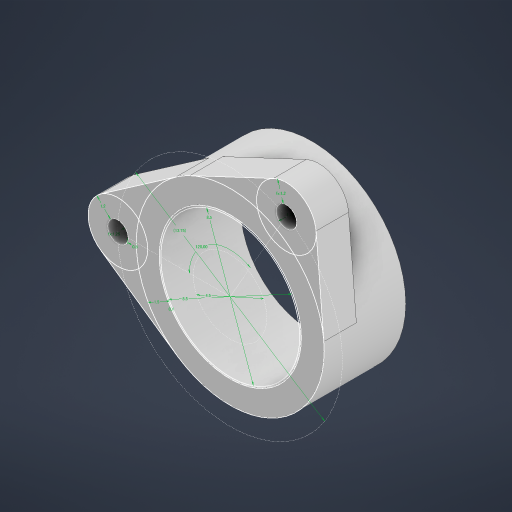
# Autodesk Inventor part: motorauxiliary
Saved by Autodesk Inventor 2023.5 (Build 275446000, 446)
## iProperties
Created: 2024-12-07
Part Number: motorauxiliary
Material: 一般
Document SubType Name: Modeling
Designer: IshiiLabHonda
Density: 1 g/cm^3
Appearance: 既定
Author: IshiiLabHonda
Autodesk Inventor part; units mm, degrees
ref_plane "YZ Plane" through (0, 0, 0) normal (1, 0, 0) x (0, 1, 0)
ref_plane "XZ Plane" through (0, 0, 0) normal (0, 1, 0) x (-1, 0, 0)
ref_plane "XY Plane" through (0, 0, 0) normal (0, 0, 1) x (1, 0, 0)
sketch "スケッチ1" plane through (0, 0, 0) normal (0, 0, 1) x (1, 0, 0)
  circle A0 centre (0, 0) radius 2.25 construction
  circle A1 centre (0, 0) radius 4.35
  circle A2 centre (0, 0) radius 5.75
  circle A3 centre (-6.875, 0) radius 0.625
  circle A4 centre (3.4375, 5.9539) radius 0.625
  circle A5 centre (0, 0) radius 6.875 construction
  circle A6 centre (-6.875, 0) radius 1.825
  circle A7 centre (3.4375, 5.9539) radius 1.825
  line L0 (-7.9169, 1.4983) -> (-3.2827, 4.7208)
  line L1 (-7.9169, -1.4983) -> (-3.2827, -4.7208)
  line L2 (5.2561, 6.1071) -> (5.7297, 0.4825)
  line L3 (-2.447, 5.2033) -> (2.6608, 7.6054)
  line L4 (3.4375, 5.9539) -> (0, 0) construction
  line L5 (0, 0) -> (-6.875, 0) construction
  circle A8 centre (0, 0) radius 4.25
  circle A9 centre (0, 0) radius 4.25
  point P0 (3.9306, 4.1968)
  point P1 (1.6692, 5.5024)
  point P2 (-5.5998, 1.3056)
  point P3 (-5.5998, -1.3056)
  dimension "d2" = 4.5
  dimension "d5" = 1.25
  dimension "d6" = 1.25
  dimension "d7" = 1.2
  dimension "d8" = 1.2
  dimension "d9" = 0.5
  dimension "d18" = 120
  dimension "d22" = 13.75
  dimension "d23" = 8.5
  dimension "d25" = 8.5
  dimension "d26" = 1.5
  dimension "d27" = 0.1
  constraints: 12 end point, 10 centre point, 10 point on circle, 9 coincident, 8 tangent, 1 horizontal
  measures "d2" diameter of A0
  measures "d5" diameter of A4
  measures "d6" diameter of A3
  measures "d7" radial gap between concentric circles of A6 A3
  measures "d8" radial gap between concentric circles of A7 A4
  measures "d18" angle of L5 L4
  measures "d22" diameter of A5
  measures "d23" diameter of A8
  measures "d25" diameter of A9
  measures "d26" radial gap between concentric circles of A2 A9
  measures "d27" radial gap between concentric circles of A1 A8
extrude "押し出し1" add sketch "スケッチ1" against normal blind 5 contours A2 A6 A7 | A7 A2 | A2 A6 picked at (2.6949, 4.8059) picked at (-5.5055, 0)
extrude "押し出し3" add sketch "スケッチ1" against normal blind 2 contours L1 A6 A2 | A6 A2 | A6 L0 A2 picked at (-5.951, -0.7528)
extrude "押し出し4" add sketch "スケッチ1" against normal blind 2 contours A2 A7 L2 | A2 A7 | A2 L3 A7 picked at (3.6121, 4.7707)
equation "\"d6\" = d5"
equation "\"d8\" = d7"
